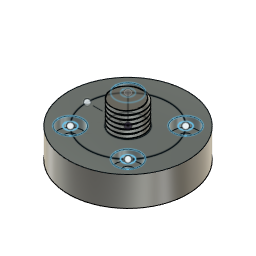
BasePlate (Autodesk Fusion 360 design; units mm, degrees)
Autodesk Fusion 360 part; units mm, degrees
note: some values were not read from the file. Set by a fixed rule: which sketch regions a step uses.
sketch "Sketch1" plane through (0, 0, 0) normal (0, 0, 1) x (1, 0, 0)
  circle A0 centre (0, 0) radius 36.5
  dimension "d56" = 73
  constraint coincident A0.centre origin
  measures "d56" diameter of A0
extrude "Extrude1" add sketch "Sketch1" along normal blind 18
sketch "Sketch2" plane through (0, 0, 18) normal (0, 0, 1) x (-1, 0, 0)
  circle A0 centre (0, 0) radius 36.5
  circle A1 centre (0, 0) radius 25
  line L0 (0, 0) -> (17.6777, -17.6777)
  line L1 (0, 0) -> (25, 0) construction
  circle A2 centre (17.6777, -17.6777) radius 7.5
  circle A3 centre (17.6777, -17.6777) radius 3.25
  circle A4 centre (17.6777, 17.6777) radius 3.25
  circle A5 centre (17.6777, 17.6777) radius 7.5
  circle A6 centre (-17.6777, 17.6777) radius 3.25
  circle A7 centre (-17.6777, 17.6777) radius 7.5
  circle A8 centre (-17.6777, -17.6777) radius 3.25
  circle A9 centre (-17.6777, -17.6777) radius 7.5
  circle A10 centre (0, 0) radius 10
  dimension "d59" = 50
  dimension "d60" = 45
  dimension "d61" = 15
  dimension "d62" = 6.5
  dimension "d64" = 360
  dimension "d69" = 20
  constraint coincident A0.centre A1.centre
  constraint horizontal L1
  constraint coincident L0.end A2.centre
  constraint concentric A2 A3
  constraint concentric A1 A10
  measures "d59" diameter of A1
  measures "d60" angle of L0 L1
  measures "d61" diameter of A2
  measures "d62" diameter of A3
  measures "d69" diameter of A10
extrude "Extrude2" cut sketch "Sketch2" against normal up to surface (18 mm away) contours A1 A4 | A1 A4 | A1 A3 | A1 L0 A3 | A1 L0 A3 | A1 A6 | A1 A6 | A1 A8 | A1 A8
extrude "Extrude3" cut sketch "Sketch2" against normal blind 6 contours A1 A4 A5 | A1 A4 A5 | A1 A2 A3 | A1 L0 A2 A3 | A1 L0 A2 A3 | A1 A6 A7 | A1 A6 A7 | A1 A8 A9 | A1 A8 A9
extrude "Extrude4" add sketch "Sketch2" along normal blind 15 contours A10
thread "Thread1" "ISO Metric profile 20.0 M20x2.5 6g" major diameter 19.7905 minor diameter 16.938 pitch 2.5 angle 60 modelled right hand crest width 0.36 on face at (-9.9876, -0.4985, 28) crest through (-9.8953, 0, 17.375)
